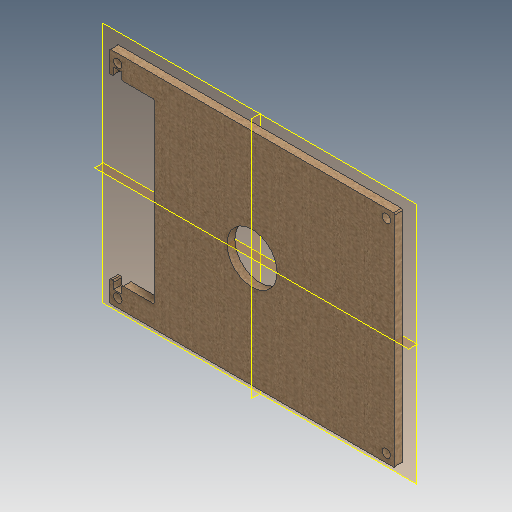
# Autodesk Inventor part: MDF_Top_Big_Mic
Saved by Autodesk Inventor 2021 (Build 250183000, 183)
## iProperties
Created: 2021-02-17
Part Number: MDF_Top_Big_Mic
Material: MDF Medium Density Fiberboard
Document SubType Name: Modeling
Designer: negt20
Density: 0.8 g/cm^3
Appearance: Cardboard - Corrugated
Author: negt20
Autodesk Inventor part; units mm, degrees
sketch "Sketch1" plane through (0, 0, 0) normal (0, 0, 1) x (1, 0, 0)
  line L0 (-109.5, 84.5) -> (109.5, 84.5)
  line L1 (109.5, 84.5) -> (109.5, -84.5)
  line L2 (109.5, -84.5) -> (-109.5, -84.5)
  line L3 (-109.5, -84.5) -> (-109.5, 84.5)
  point P0 (0, 84.5)
  point P1 (0, 0)
  point P2 (-109.5, 0)
  dimension "d0" = 219
  dimension "d1" = 169
  constraints: 8 end point, 2 midpoint, 2 parallel, 1 horizontal, 1 horizontal alignment, 1 perpendicular, 1 vertical alignment
  measures "d0" distance of L1.end L2.end
  measures "d1" distance of L0.end L1.end
extrude "Extrusion1" add sketch "Sketch1" along normal blind 6
sketch "Sketch2" plane through (0, 0, 6) normal (0, 0, 1) x (1, 0, 0)
  line L0 (-103, -84.5) -> (-103, -78) construction
  circle A0 centre (-103, -78) radius 3.25
  line L1 (-103, -78) -> (-103, -74) construction
  line L2 (-106.25, -68) -> (-99.75, -68)
  line L3 (-99.75, -68) -> (-99.75, -74)
  line L4 (-99.75, -74) -> (-106.25, -74)
  line L5 (-106.25, -74) -> (-106.25, -68)
  line L6 (-109.5, -84.5) -> (-103, -84.5) construction
  point P0 (0, 0)
  dimension "d38" = 6.5
  dimension "d39" = 6.5
  dimension "d44" = 4
  dimension "d45" = 6.5
  dimension "d46" = 6
  dimension "d58" = 6.5
  constraints: 14 end point, 3 coincident, 2 parallel, 1 centre point, 1 horizontal, 1 midpoint, 1 perpendicular, 1 vertical
  measures "d38" distance of L0.start L0.end
  measures "d39" diameter of A0
  measures "d44" distance of L1.start L1.end
  measures "d45" distance of L3.end L4.end
  measures "d46" distance of L2.end L3.end
  measures "d58" distance of L6.start L0.start
extrude "Extrusion2" cut sketch "Sketch2" against normal blind 6 contours A0
mirror "Mirror3" about plane through (0, 0, 0) normal (1, 0, 0) of "Extrusion2"
mirror "Mirror7" about plane through (0, 0, 0) normal (0, 1, 0) of "Extrusion2", "Mirror3"
sketch "Sketch7" plane through (0, 0, 6) normal (0, 0, 1) x (1, 0, 0)
  line L0 (-109.5, 84.5) -> (-109.5, -84.5) projected
  line L1 (-109.5, 68) -> (-75, 68)
  line L2 (-75, 68) -> (-75, -68)
  line L3 (-75, -68) -> (-109.5, -68)
  line L4 (-109.5, -68) -> (-109.5, 68)
  point P0 (0, 0)
  point P1 (-109.5, 0)
  point P2 (-109.5, 0)
  dimension "d40" = 34.5
  dimension "d41" = 136
  constraints: 8 end point, 2 midpoint, 2 parallel, 1 coincident, 1 horizontal, 1 perpendicular, 1 point on line
  measures "d40" distance of L2.end L3.end
  measures "d41" distance of L1.end L2.end
extrude "Extrusion6" cut sketch "Sketch7" against normal blind 10
sketch "Sketch8" plane through (0, 0, 6) normal (0, 0, 1) x (1, 0, 0)
  circle A0 centre (-103, -78) radius 3.25 projected
  line L0 (-103, -78) -> (-103, -73.75) construction
  line L1 (-106.125, -68) -> (-99.875, -68)
  line L2 (-99.875, -68) -> (-99.875, -73.75)
  line L3 (-99.875, -73.75) -> (-106.125, -73.75)
  line L4 (-106.125, -73.75) -> (-106.125, -68)
  point P0 (0, 0)
  dimension "d47" = 4.25
  dimension "d48" = 6.25
  dimension "d49" = 5.75
  constraints: 10 end point, 2 coincident, 2 parallel, 1 horizontal, 1 midpoint, 1 perpendicular, 1 vertical
  measures "d47" distance of L0.start L0.end
  measures "d48" distance of L2.end L3.end
  measures "d49" distance of L1.end L2.end
extrude "Extrusion7" cut sketch "Sketch8" against normal blind 6 contours L1 L2 L3 L4
mirror "Mirror8" about plane through (0, 0, 0) normal (0, 1, 0) of "Extrusion7"
fillet "Fillet5" radius 1 12 edges at (-109.5, -84.5, 3) (109.5, -84.5, 3) (-75, -68, 3) (109.5, 84.5, 3) (-109.5, 84.5, 3) (-109.5, 68, 3) (-75, 68, 3) (-99.875, 68, 3) (-106.125, 68, 3) (-99.875, -68, 3) (-109.5, -68, 3) (-106.125, -68, 3)
sketch "Sketch9" plane through (0, 0, 6) normal (0, 0, 1) x (1, 0, 0)
  line L0 (-75, 44.5) -> (39, 44.5) construction
  line L1 (39, 44.5) -> (39, -44.5) construction
  line L2 (39, -44.5) -> (-75, -44.5) construction
  line L3 (-75, -44.5) -> (-75, 44.5) construction
  line L4 (-75, 67) -> (-75, -67) projected
  line L5 (39, 44.5) -> (-75, -44.5) construction
  circle A0 centre (0, 0) radius 19.25
  point P0 (-75, 0)
  point P1 (-75, 0)
  point P2 (-75, 0)
  dimension "d53" = 114
  dimension "d54" = 89
  dimension "d55" = 38.5
  constraints: 10 end point, 3 coincident, 3 midpoint, 2 parallel, 1 centre point, 1 horizontal, 1 perpendicular
  measures "d53" distance of L1.end L2.end
  measures "d54" distance of L0.end L1.end
  measures "d55" diameter of A0
extrude "Extrusion8" cut sketch "Sketch9" against normal through all
equation "\"d7\" = d46"
body "Solid1"
